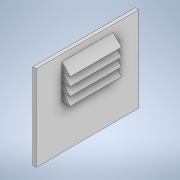
# Autodesk Inventor part: Part1
Saved by Autodesk Inventor 2022.6 (Build 266554010, 554A)
## iProperties
Created: 2025-03-19
Part Number: Part1
Material: Generic
Document SubType Name: Modeling
Designer: khinm
Density: 1 g/cm^3
Appearance: Default
Author: khinm
Autodesk Inventor part; units mm, degrees
ref_plane "YZ Plane" through (0, 0, 0) normal (1, 0, 0) x (0, 1, 0)
ref_plane "XZ Plane" through (0, 0, 0) normal (0, 1, 0) x (-1, 0, 0)
sketch "Sketch1" plane through (0, 0, 0) normal (1, 0, 0) x (0, 1, 0)
  line L0 (0, 76.2) -> (127, 76.2)
  line L1 (127, 76.2) -> (127, -76.2)
  line L2 (127, -76.2) -> (0, -76.2)
  line L3 (0, -76.2) -> (0, 76.2)
  point P0 (0, 0)
  point P1 (0, 0)
  dimension "d0" = 127
  dimension "d1" = 152.4
  constraints: 8 end point, 2 parallel, 1 coincident, 1 horizontal, 1 midpoint, 1 perpendicular
  measures "d0" distance of L1.end L2.end
  measures "d1" distance of L0.end L1.end
extrude "Extrusion1" add sketch "Sketch1" along normal blind 5.08
sketch "Sketch11" plane through (0, 0, 0) normal (0, 0, 1) x (1, 0, 0)
  line L0 (5.08, 127) -> (5.08, 0) projected
  line L1 (5.08, 0) -> (5.08, 127) projected
  line L2 (5.08, 116.84) -> (5.08, 104.14)
  line L3 (5.08, 104.14) -> (17.78, 104.14)
  line L4 (17.78, 104.14) -> (5.08, 116.84)
  line L5 (0, 127) -> (5.08, 127) projected
  point P0 (0, 0)
  point P1 (2.54, 127)
  dimension "d31" = 10.16
  dimension "d32" = 12.7
  dimension "d33" = 45
  constraints: 6 end point, 2 point on line, 1 horizontal, 1 midpoint
  measures "d31" vertical distance of L2.start point (2.54, 127)
  measures "d32" distance of L2.end L2.start
  measures "d33" angle of L4 L0
extrude "Extrusion5" add sketch "Sketch11" along normal mid plane 76.2
ref_plane "Work Plane5" through (0, 0, 0) normal (0, 0, 1) x (1, 0, 0)
sketch "Sketch17" plane through (0, 0, 0) normal (0, 0, 1) x (1, 0, 0)
  line L0 (0, 0) -> (0, 127) projected
  line L1 (17.78, 104.14) -> (5.08, 104.14) projected
  line L2 (15.24, 104.14) -> (0, 104.14)
  line L3 (0, 114.3) -> (5.08, 114.3)
  line L4 (5.08, 0) -> (5.08, 127) projected
  line L5 (5.08, 114.3) -> (15.24, 104.14)
  line L6 (0, 104.14) -> (0, 114.3)
  dimension "d45" = 10.16
  dimension "d46" = 45
  constraints: 8 end point, 4 point on line, 1 collinear, 1 parallel, 1 perpendicular
  measures "d45" distance from line of L2 L3.start
  measures "d46" angle of L5 L1
extrude "Extrusion6" cut sketch "Sketch17" along normal mid plane 71.12
pattern_linear "Rectangular Pattern4" count 4 spacing 12.7 along (0, -1, 0) of "Extrusion5", "Extrusion6"
body "Solid1"
